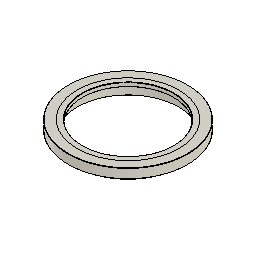
Top Teflon PLA Ring v2 (Autodesk Fusion 360 design; units mm, degrees)
Autodesk Fusion 360 part; units mm, degrees
sketch "Sketch1" plane through (0, 0, 0) normal (0, 0, 1) x (1, 0, 0)
  circle A0 centre (0, 0) radius 89
  dimension "d1" = 178
  constraint coincident A0.centre origin
  measures "d1" diameter of A0
extrude "Extrude1" add sketch "Sketch1" along normal blind 14.2748
sketch "Sketch2" plane through (0, 0, 0) normal (0, 0, -1) x (1, 0, 0)
  circle A0 centre (0, 0) radius 89
  circle A1 centre (0, 0) radius 78.125
  circle A2 centre (0, 0) radius 75.6231
  dimension "d4" = 156.25
  dimension "d5" = 151.2462
  constraint coincident A0.centre A1.centre
  constraint concentric A1 A2
  measures "d4" diameter of A1
  measures "d5" diameter of A2
extrude "Extrude2" add sketch "Sketch2" along normal blind 8.255 contours A1
extrude "Extrude3" cut 1 faces at (17.6402, 5.9585, 0) along direction (0, 0, 1) blind 60
sketch "Sketch3" plane through (0, 0, 0) normal (0, 0, -1) x (1, 0, 0)
  circle A0 centre (0, 0) radius 75.6231
  circle A1 centre (0, 0) radius 67.625
  dimension "d10" = 135.25
  constraint concentric A0 A1
  measures "d10" diameter of A1
extrude "Extrude4" add sketch "Sketch3" against normal blind 14.275
extrude "Extrude5" cut 1 faces at (72.4237, 7.1167, 0) along direction (0, 0, 1) blind 6
extrude "Extrude6" cut 1 faces at (72.4237, 7.1167, 6) along direction (0, 0, 1) blind 2.255
fillet "Fillet1" radius 1 1 edges at (-72.8381, -28.2512, 0)
fillet "Fillet2" radius 0.5 1 edges at (-70.5055, -27.3465, -8.255)
fillet "Fillet3" radius 0.5 1 edges at (-72.8381, 28.2512, -8.255)
fillet "Fillet4" radius 0.5 1 edges at (-70.5055, -27.3465, 8.255)
fillet "Fillet5" radius 0.5 1 edges at (-82.9771, -32.1838, 0)
fillet "Fillet6" radius 0.5 1 edges at (-82.9771, -32.1838, 14.2748)
fillet "Fillet7" radius 0.5 2 edges at (-63.0486, 24.4542, 14.275) (-63.0486, 24.4542, 8.255)
equation "d2 = 0.27 in + 0.292 in"
equation "d5 = d4 - 0.197 in"
equation "d6 = 0.625 in - 0.3 in"
equation "d15 = 6.00 mm - 0.325 in"
